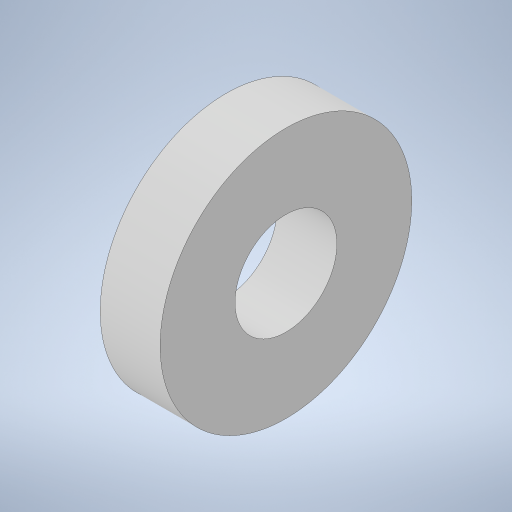
# Autodesk Inventor part: elbow_upperplate_left_spacer
Saved by Autodesk Inventor 2024 (Build 280153000, 153)
## iProperties
Created: 2025-08-07
Part Number: elbow_upperplate_left_spacer
Material: 一般
Document SubType Name: Modeling
Designer: HosodaLab2
Density: 1 g/cm^3
Appearance: 既定
Author: HosodaLab2
Autodesk Inventor part; units mm, degrees
ref_plane "YZ Plane" through (0, 0, 0) normal (1, 0, 0) x (0, 1, 0)
ref_plane "XZ Plane" through (0, 0, 0) normal (0, 1, 0) x (-1, 0, 0)
ref_plane "XY Plane" through (0, 0, 0) normal (0, 0, 1) x (1, 0, 0)
sketch "スケッチ1" plane through (0, 0, 0) normal (0, 1, 0) x (-1, 0, 0)
  circle A0 centre (0, 0) radius 4.25
  circle A1 centre (0, 0) radius 10.5
  dimension "d0" = 8.5
  dimension "d1" = 21
  constraints: 2 centre point, 2 coincident
  measures "d0" diameter of A0
  measures "d1" diameter of A1
extrude "押し出し1" add sketch "スケッチ1" along normal blind 5
